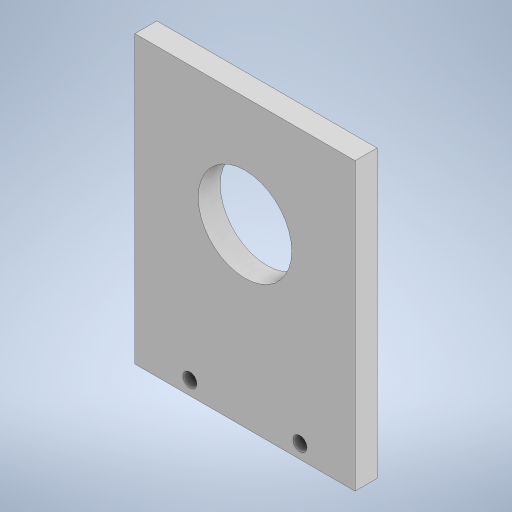
# Autodesk Inventor part: FloorMountFacePlate
Saved by Autodesk Inventor 2024 (Build 280153000, 153)
## iProperties
Created: 2024-02-13
Part Number: FloorMountFacePlate
Material: Generic
Document SubType Name: Modeling
Designer: yusuf
Density: 1 g/cm^3
Appearance: Default
Author: yusuf
Autodesk Inventor part; units mm, degrees
ref_plane "YZ Plane" through (0, 0, 0) normal (1, 0, 0) x (0, 1, 0)
ref_plane "XZ Plane" through (0, 0, 0) normal (0, 1, 0) x (-1, 0, 0)
ref_plane "XY Plane" through (0, 0, 0) normal (0, 0, 1) x (1, 0, 0)
sketch "Sketch1" plane through (0, 0, 0) normal (0, 0, 1) x (1, 0, 0)
  line L0 (0, 0) -> (200, 0)
  line L1 (200, 0) -> (200, 260)
  line L2 (200, 260) -> (0, 260)
  line L3 (0, 260) -> (0, 0)
  dimension "d0" = 200
  dimension "d1" = 260
  constraints: 8 end point, 2 parallel, 1 horizontal, 1 perpendicular
  measures "d0" distance of L1.end L2.end
  measures "d1" distance of L0.end L1.end
extrude "Extrusion1" add sketch "Sketch1" along normal blind 20
sketch "Sketch2" plane through (0, 0, 20) normal (0, 0, 1) x (1, 0, 0)
  circle A0 centre (100, 160) radius 42.5
  line L0 (200, 260) -> (0, 260) projected
  line L1 (0, 260) -> (0, 0) projected
  dimension "d4" = 85
  dimension "d5" = 100
  dimension "d6" = 100
  constraints: 1 centre point
  measures "d4" diameter of A0
  measures "d5" distance from line of L0 A0.centre
  measures "d6" distance from line of L1 A0.centre
extrude "Extrusion2" cut sketch "Sketch2" against normal blind 20
sketch "Sketch3" plane through (0, 0, 0) normal (0, 0, -1) x (-1, 0, 0)
  circle A0 centre (-150, 12.5) radius 6.35
  circle A1 centre (-50, 12.5) radius 6.35
  line L0 (0, 0) -> (-200, 0) projected
  line L1 (-200, 0) -> (-200, 260) projected
  line L2 (0, 260) -> (0, 0) projected
  dimension "d9" = 12.7
  dimension "d10" = 12.7
  dimension "d11" = 12.5
  dimension "d12" = 12.5
  dimension "d13" = 50
  dimension "d14" = 50
  constraints: 2 centre point
  measures "d9" diameter of A0
  measures "d10" diameter of A1
  measures "d11" distance from line of L0 A0.centre
  measures "d12" distance from line of L0 A1.centre
  measures "d13" distance from line of L1 A0.centre
  measures "d14" distance from line of L2 A1.centre
extrude "Extrusion3" cut sketch "Sketch3" against normal blind 20
equation "\"d12\" = d11"
equation "\"d14\" = d13"
body "Solid1"
